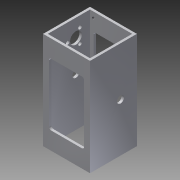
# Autodesk Inventor part: Gear box改
Saved by Autodesk Inventor 2015 (Build 190159000, 159)
## iProperties
Created: 2015-05-20
Part Number: Gear box改
Material: アルミニウム
Document SubType Name: Modeling
Designer: kenta
Density: 2.7 g/cm^3
Appearance: サテン
Mass: 50.0415 g
Surface Area: 200.498 cm^2
Volume: 18.5339 cm^3
Author: kenta
Autodesk Inventor part; units mm, degrees
note: some values were not read from the file. Chosen so that the rebuilt part matches the saved one: direction of "穴1".
ref_plane "YZ Plane" through (0, 0, 0) normal (1, 0, 0) x (0, 1, 0)
ref_plane "XZ Plane" through (0, 0, 0) normal (0, 1, 0) x (-1, 0, 0)
ref_plane "XY Plane" through (0, 0, 0) normal (0, 0, 1) x (1, 0, 0)
sketch "スケッチ1" plane through (0, 0, 0) normal (0, 0, 1) x (1, 0, 0)
  line L0 (-20, 20) -> (20, 20)
  line L1 (20, 20) -> (20, -20)
  line L2 (20, -20) -> (-20, -20)
  line L3 (-20, -20) -> (-20, 20)
  line L4 (-20, 20) -> (20, -20) construction
  line L5 (20, 20) -> (-20, -20) construction
  line L6 (-18, 18) -> (18, 18)
  line L7 (18, 18) -> (18, -18)
  line L8 (18, -18) -> (-18, -18)
  line L9 (-18, -18) -> (-18, 18)
  line L10 (-18, 18) -> (18, -18) construction
  line L11 (18, 18) -> (-18, -18) construction
  point P0 (0, 0)
  point P1 (0, 0)
  dimension "d0" = 40
  dimension "d1" = 40
  dimension "d2" = 2
  dimension "d3" = 2
  constraints: 24 end point, 6 midpoint, 4 parallel, 2 horizontal, 2 perpendicular
  measures "d0" distance of L1.end L2.end
  measures "d1" distance of L0.end L1.end
  measures "d2" distance between parallel lines of L8 L2
  measures "d3" distance between parallel lines of L1 L7
extrude "押し出し1" add sketch "スケッチ1" along normal blind 83
sketch "スケッチ3" plane through (-20, 20, 0) normal (0, 1, 0) x (1, 0, 0)
  line L0 (5, -68) -> (35, -68)
  line L1 (35, -68) -> (35, -15)
  line L2 (35, -15) -> (5, -15)
  line L3 (5, -15) -> (5, -68)
  line L4 (40, -83) -> (0, -83) projected
  line L5 (0, 0) -> (40, 0) projected
  line L6 (40, 0) -> (40, -83) projected
  line L7 (0, 0) -> (0, -83) projected
  point P0 (20, 0)
  dimension "d6" = 15
  dimension "d7" = 15
  dimension "d8" = 5
  dimension "d9" = 5
  constraints: 8 end point, 2 parallel, 1 horizontal, 1 perpendicular
  measures "d6" distance between parallel lines of L4 L0
  measures "d7" distance between parallel lines of L5 L2
  measures "d8" distance between parallel lines of L6 L1
  measures "d9" distance between parallel lines of L7 L3
extrude "押し出し2" cut sketch "スケッチ3" against normal blind 100 contours L3 L2 L1 L0
fillet "フィレット1" radius 2 8 edges at (-15, 19, 68) (-15, 19, 15) (15, 19, 15) (15, 19, 68) (15, -19, 68) (-15, -19, 68) (-15, -19, 15) (15, -19, 15)
sketch "スケッチ4" plane through (-20, 20, 0) normal (0, 1, 0) x (1, 0, 0)
  line L0 (0, 0) -> (0, -83) projected
  line L1 (0, 0) -> (40, 0) projected
  line L2 (40, 0) -> (40, -83) projected
  line L3 (40, -83) -> (0, -83) projected
  point P0 (20, 0)
  point P1 (5, -5)
  point P2 (5, -78)
  point P3 (35, -78)
  point P4 (35, -5)
  dimension "d13" = 5
  dimension "d14" = 5
  dimension "d15" = 5
  dimension "d16" = 5
  dimension "d17" = 5
  dimension "d18" = 5
  dimension "d19" = 5
  dimension "d20" = 5
  measures "d13" distance from line of L0 point (5, -5)
  measures "d14" distance from line of point (5, -5) L1
  measures "d15" distance from line of point (35, -5) L1
  measures "d16" distance from line of L2 point (35, -5)
  measures "d17" distance from line of point (35, -78) L2
  measures "d18" distance from line of point (35, -78) L3
  measures "d19" distance from line of point (5, -78) L3
  measures "d20" distance from line of L0 point (5, -78)
hole "穴1" at (-15, 20, 5) at (-15, 20, 78) at (15, 20, 78) at (15, 20, 5) direction (0, -1, 0) diameter 2.5 end up to surface
thread "ねじ1" size "M2.5x0.45" class "6H" standard "ANSI Metric M Profile" full length
thread "ねじ2" size "M2.5x0.45" class "6H" standard "ANSI Metric M Profile" full length
thread "ねじ3" size "M2.5x0.45" class "6H" standard "ANSI Metric M Profile" full length
thread "ねじ4" size "M2.5x0.45" class "6H" standard "ANSI Metric M Profile" full length
sketch "スケッチ6" plane through (-20, -20, 0) normal (-1, 0, 0) x (0, 0, 1)
  line L0 (0, 0) -> (0, 40) projected
  line L1 (0, 40) -> (83, 40) projected
  line L2 (83, 40) -> (83, 0) projected
  point P0 (0, 20)
  point P1 (68, 26)
  dimension "d46" = 14
  dimension "d54" = 15
  measures "d46" distance from line of point (68, 26) L1
  measures "d54" distance from line of L2 point (68, 26)
hole "穴3" at (-20, 6, 68) direction (1, 0, 0) diameter 10 depth 8
sketch "スケッチ7" plane through (-20, -20, 0) normal (-1, 0, 0) x (0, 0, 1)
  line L0 (0, 40) -> (83, 40) projected
  line L1 (83, 40) -> (83, 0) projected
  point P0 (0, 20)
  point P1 (68, 19)
  dimension "d55" = 21
  dimension "d56" = 15
  measures "d55" distance from line of point (68, 19) L0
  measures "d56" distance from line of L1 point (68, 19)
hole "穴4" at (-20, -1, 68) direction (1, 0, 0) diameter 3 depth 8
pattern_circular "円形状パターン1" count 3 over 360 about axis through (-16, 6, 68) along (-1, 0, 0) of "穴4"
sketch "スケッチ8" plane through (-20, -20, 0) normal (-1, 0, 0) x (0, 0, 1)
  line L0 (83, 40) -> (83, 0) projected
  line L1 (0, 0) -> (83, 0) projected
  line L2 (0, 40) -> (83, 40) projected
  circle A0 centre (68, 26) radius 5 projected
  point P0 (0, 20)
  point P1 (41.5, 26)
  dimension "d77" = 14
  dimension "d78" = 26.5
  measures "d77" distance from line of point (41.5, 26) L2
  measures "d78" distance of A0.centre point (41.5, 26)
hole "穴5" at (-20, 6, 41.5) direction (1, 0, 0) diameter 6 end through all
